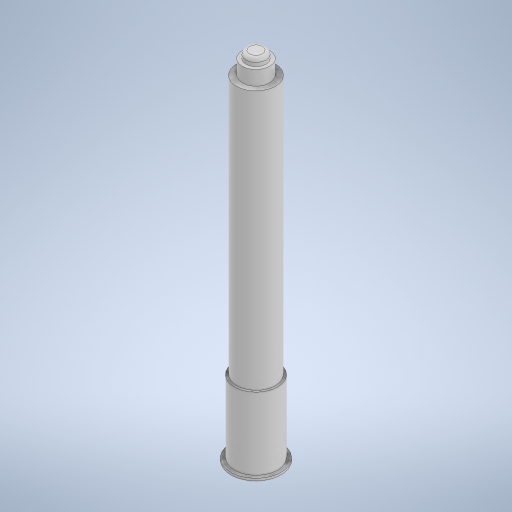
# Autodesk Inventor part: middle shaft
Saved by Autodesk Inventor 2023 (Build 270158030, 158C)
## iProperties
Created: 2023-03-03
Part Number: middle shaft
Material: Generic
Document SubType Name: Modeling
Designer: mpino
Density: 1 g/cm^3
Appearance: Default
Author: mpino
Autodesk Inventor part; units mm, degrees
ref_plane "YZ Plane" through (0, 0, 0) normal (1, 0, 0) x (0, 1, 0)
ref_plane "XZ Plane" through (0, 0, 0) normal (0, 1, 0) x (-1, 0, 0)
ref_plane "XY Plane" through (0, 0, 0) normal (0, 0, 1) x (1, 0, 0)
sketch "Sketch1" plane through (0, 0, 0) normal (0, 1, 0) x (-1, 0, 0)
  circle A0 centre (0, 0) radius 22.225
  dimension "d0" = 44.45
  constraints: 1 centre point, 1 coincident
  measures "d0" diameter of A0
extrude "Extrusion1" add sketch "Sketch1" along normal blind 3.175
fillet "Fillet1" radius 1.27 1 edges at (22.225, 0, 0)
sketch "Sketch2" plane through (0, 3.175, 0) normal (0, 1, 0) x (1, 0, 0)
  circle A0 centre (0, 0) radius 19.05
  dimension "d4" = 38.1
  constraints: 1 centre point, 1 coincident
  measures "d4" diameter of A0
extrude "Extrusion2" add sketch "Sketch2" along normal blind 63.5
sketch "Sketch3" plane through (0, 66.675, 0) normal (0, 1, 0) x (1, 0, 0)
  circle A0 centre (0, 0) radius 17.145
  dimension "d7" = 34.29
  constraints: 1 centre point, 1 coincident
  measures "d7" diameter of A0
extrude "Extrusion3" add sketch "Sketch3" along normal blind 228.6
sketch "Sketch4" plane through (0, 295.275, 0) normal (0, 1, 0) x (1, 0, 0)
  circle A0 centre (0, 0) radius 12.065
  dimension "d10" = 24.13
  constraints: 1 centre point, 1 coincident
  measures "d10" diameter of A0
extrude "Extrusion4" add sketch "Sketch4" along normal blind 12.7
sketch "Sketch5" plane through (0, 307.975, 0) normal (0, 1, 0) x (1, 0, 0)
  circle A0 centre (0, 0) radius 8.89
  dimension "d14" = 17.78
  constraints: 1 centre point, 1 coincident
  measures "d14" diameter of A0
extrude "Extrusion5" add sketch "Sketch5" along normal blind 6.35
fillet "Fillet3" radius 3.175 1 edges at (-8.89, 314.325, 0)
body "Solid1"
